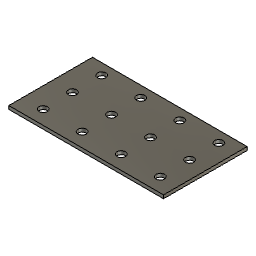
plate v1 (Autodesk Fusion 360 design; units mm, degrees)
Autodesk Fusion 360 part; units mm, degrees
box "BoxPrimitive1" add length 100 width 185 height 4 placed x (0, -1, 0) y (1, 0, 0) z (0, 0, 1) at (-207.7492, 131.2779, 0)
sketch "Sketch2" plane through (0, 0, 4) normal (0, 0, 1) x (-1, 0, 0)
  line L0 (207.7492, -31.2779) -> (22.7492, -31.2779)
  line L1 (22.7492, -31.2779) -> (22.7492, -131.2779)
  line L2 (22.7492, -131.2779) -> (207.7492, -131.2779)
  line L3 (207.7492, -131.2779) -> (207.7492, -31.2779)
  circle A0 centre (43.5078, -48.1327) radius 5
  circle A1 centre (90.1744, -48.1327) radius 5
  circle A2 centre (136.8411, -48.1327) radius 5
  circle A3 centre (183.5078, -48.1327) radius 5
  circle A4 centre (43.5078, -83.1327) radius 5
  circle A5 centre (43.5078, -118.1327) radius 5
  circle A6 centre (90.1744, -83.1327) radius 5
  circle A7 centre (136.8411, -83.1327) radius 5
  circle A8 centre (183.5078, -83.1327) radius 5
  circle A9 centre (90.1744, -118.1327) radius 5
  circle A10 centre (136.8411, -118.1327) radius 5
  circle A11 centre (183.5078, -118.1327) radius 5
  dimension "d7" = 10
  dimension "d10" = 140
  dimension "d11" = 0
  dimension "d14" = 0
  dimension "d15" = -70
  dimension "d18" = 140
  dimension "d19" = 0
  dimension "d22" = 140
  dimension "d23" = 0
  measures "d7" diameter of A0
extrude "Extrude1" cut sketch "Sketch2" against normal blind 5 contours A0 | A1 | A2 | A3 | A4 | A5 | A6 | A7 | A8 | A9 | A10 | A11
